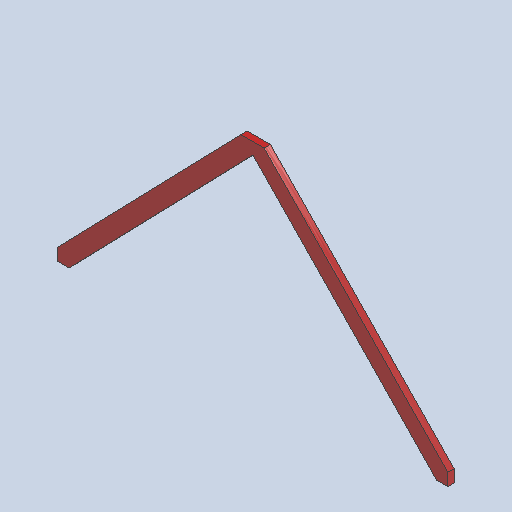
# Autodesk Inventor part: 48x2x4-2
Saved by Autodesk Inventor 2025.1 (Build 291241020, 241B)
## iProperties
Created: 2024-09-20
Part Number: 48x2x4-2
Material: Generic
Document SubType Name: Modeling
Designer: User
Density: 1 g/cm^3
Appearance: Default
Stock Number: 6x2
Author: User
Autodesk Inventor part; units mm, degrees
ref_plane "YZ Plane" through (0, 0, 0) normal (1, 0, 0) x (0, 1, 0)
ref_plane "XZ Plane" through (0, 0, 0) normal (0, 1, 0) x (-1, 0, 0)
ref_plane "XY Plane" through (0, 0, 0) normal (0, 0, 1) x (1, 0, 0)
sketch "Sketch1" plane through (0, 0, 0) normal (0, 0, 1) x (1, 0, 0)
  line L0 (0, 0) -> (-2438.4, 0) projected
  line L1 (-38.1, 0) -> (-38.1, -1219.2) projected
  line L2 (0, -1219.2) -> (-2438.4, -1219.2) projected
  line L3 (-2400.3, 0) -> (-2400.3, -1219.2) projected
  line L4 (-2400.3, -1219.2) -> (-2400.3, -1144.1906)
  line L5 (-2400.3, -1144.1906) -> (-1291.8653, 0)
  line L6 (-1219.2, 0) -> (-1291.8653, 0)
  line L7 (-1219.2, -70.3945) -> (-2332.1053, -1219.2)
  line L8 (-2332.1053, -1219.2) -> (-2400.3, -1219.2)
  line L9 (-1219.2, -70.3945) -> (-106.2947, -1219.2)
  line L10 (-38.1, -1219.2) -> (-106.2947, -1219.2)
  line L11 (-38.1, -1219.2) -> (-38.1, -1144.1906)
  line L12 (-38.1, -1144.1906) -> (-1151.0053, 0)
  line L13 (-1219.2, 0) -> (-1151.0053, 0)
  constraints: 20 end point, 7 point on line, 2 collinear, 2 perpendicular, 1 midpoint, 1 parallel, 2 other
extrude "Extrusion1" add sketch "Sketch1" against normal blind 38.1 contours L12 L1 L2 L9 L7 L3 L5 L0
body "Solid1"
